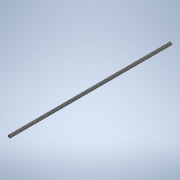
# Autodesk Inventor part: 8mm carbon fiber rod
Saved by Autodesk Inventor 2020.4 (Build 244396000, 396)
## iProperties
Created: 2021-03-19
Part Number: 8mm carbon fiber rod
Material: CFRP
Document SubType Name: Modeling
Designer: AOB
Mass: 14.2142 g
Surface Area: 199.24 cm^2
Volume: 9.94 cm^3
Density: 1.43 g/cm^3
Appearance: Carbon Fiber
Author: AOB
Autodesk Inventor part; units mm, degrees
ref_plane "YZ Plane" through (0, 0, 0) normal (1, 0, 0) x (0, 1, 0)
ref_plane "XZ Plane" through (0, 0, 0) normal (0, 1, 0) x (-1, 0, 0)
ref_plane "XY Plane" through (0, 0, 0) normal (0, 0, 1) x (1, 0, 0)
sketch "Sketch1" plane through (0, 0, 0) normal (0, 0, 1) x (1, 0, 0)
  circle A0 centre (0, 0) radius 4
  circle A1 centre (0, 0) radius 3
  dimension "d0" = 8
  dimension "d1" = 6
  constraints: 2 centre point, 2 coincident
  measures "d0" diameter of A0
  measures "d1" diameter of A1
extrude "Extrusion1" add sketch "Sketch1" along normal blind 452
body "Solid1"
